Autodesk Fusion 360 part; units mm, degrees
(part 5 of 6)
  spline S26 degree 5 poles (0.4699, -23.4876) (0.4701, -23.4979) (0.4708, -23.5184) (0.4725, -23.5492) (0.4763, -23.5901) (0.4831, -23.6411) (0.4912, -23.692) (0.5002, -23.7429) (0.5098, -23.7937) (0.5196, -23.8445) (0.5298, -23.8953) (0.5405, -23.9461) (0.5517, -23.9968) (0.5636, -24.0474) (0.5762, -24.098) (0.5894, -24.1485) (0.6032, -24.1989) (0.6175, -24.2493) (0.6321, -24.2997) (0.6472, -24.35) (0.6626, -24.4003) (0.6784, -24.4505) (0.6946, -24.5006) (0.7112, -24.5507) (0.7283, -24.6008) (0.7458, -24.6508) (0.7636, -24.7007) (0.7819, -24.7506) (0.8005, -24.8004) (0.8194, -24.8502) (0.8387, -24.8999) (0.8583, -24.9496) (0.8782, -24.9992) (0.8985, -25.0487) (0.9191, -25.0982) (0.9401, -25.1476) (0.9614, -25.197) (0.983, -25.2463) (1.0049, -25.2956) (1.0272, -25.3448) (1.0497, -25.3939) (1.0725, -25.443) (1.0957, -25.492) (1.1191, -25.5409) (1.1429, -25.5898) (1.1669, -25.6386) (1.1912, -25.6874) (1.2158, -25.7361) (1.2407, -25.7847) (1.2659, -25.8333) (1.2913, -25.8818) (1.317, -25.9303) (1.343, -25.9787) (1.3693, -26.027) (1.3958, -26.0752) (1.4226, -26.1234) (1.4497, -26.1715) (1.477, -26.2196) (1.5046, -26.2675) (1.5325, -26.3154) (1.5606, -26.3633) (1.589, -26.4111) (1.6176, -26.4588) (1.6465, -26.5064) (1.6756, -26.5539) (1.705, -26.6014) (1.7346, -26.6489) (1.7645, -26.6962) (1.7946, -26.7435) (1.8249, -26.7907) (1.8555, -26.8378) (1.8802, -26.8754) (1.8988, -26.9036) (1.9113, -26.9224) (1.9175, -26.9318) knots 0 0 0 0 0 0 0.01428571 0.02857143 0.04285714 0.05714286 0.07142857 0.08571429 0.1 0.11428571 0.12857143 0.14285714 0.15714286 0.17142857 0.18571429 0.2 0.21428571 0.22857143 0.24285714 0.25714286 0.27142857 0.28571429 0.3 0.31428571 0.32857143 0.34285714 0.35714286 0.37142857 0.38571429 0.4 0.41428571 0.42857143 0.44285714 0.45714286 0.47142857 0.48571429 0.5 0.51428571 0.52857143 0.54285714 0.55714286 0.57142857 0.58571429 0.6 0.61428571 0.62857143 0.64285714 0.65714286 0.67142857 0.68571429 0.7 0.71428571 0.72857143 0.74285714 0.75714286 0.77142857 0.78571429 0.8 0.81428571 0.82857143 0.84285714 0.85714286 0.87142857 0.88571429 0.9 0.91428571 0.92857143 0.94285714 0.95714286 0.97142857 0.98571429 1 1 1 1 1 1
  arc A60 (1.9175, -26.9318) -> (3.3501, -26.7914) centre (0, 0) ccw
  spline S27 degree 5 poles (3.3501, -26.7914) (3.3544, -26.7809) (3.363, -26.7601) (3.3757, -26.7288) (3.3926, -26.6871) (3.4135, -26.6349) (3.4341, -26.5827) (3.4545, -26.5305) (3.4746, -26.4783) (3.4944, -26.426) (3.514, -26.3737) (3.5333, -26.3214) (3.5524, -26.269) (3.5712, -26.2167) (3.5898, -26.1643) (3.6081, -26.1119) (3.6261, -26.0595) (3.6438, -26.0071) (3.6613, -25.9547) (3.6785, -25.9022) (3.6955, -25.8497) (3.7121, -25.7972) (3.7285, -25.7448) (3.7446, -25.6922) (3.7604, -25.6397) (3.776, -25.5872) (3.7912, -25.5347) (3.8062, -25.4821) (3.8209, -25.4296) (3.8352, -25.377) (3.8493, -25.3244) (3.8631, -25.2719) (3.8766, -25.2193) (3.8898, -25.1667) (3.9027, -25.1142) (3.9152, -25.0616) (3.9275, -25.009) (3.9394, -24.9564) (3.951, -24.9039) (3.9623, -24.8513) (3.9733, -24.7987) (3.9839, -24.7462) (3.9942, -24.6936) (4.0041, -24.6411) (4.0137, -24.5886) (4.023, -24.5361) (4.0319, -24.4836) (4.0404, -24.4311) (4.0486, -24.3786) (4.0564, -24.3261) (4.0639, -24.2737) (4.0709, -24.2213) (4.0775, -24.1689) (4.0837, -24.1166) (4.0894, -24.0642) (4.0948, -24.012) (4.0997, -23.9597) (4.1043, -23.9074) (4.1085, -23.8552) (4.1122, -23.8031) (4.1154, -23.7509) (4.118, -23.6989) (4.1198, -23.6469) (4.121, -23.595) (4.1216, -23.5431) (4.1217, -23.4913) (4.1215, -23.4396) (4.121, -23.3879) (4.12, -23.3362) (4.1181, -23.2847) (4.1147, -23.2334) (4.1105, -23.1925) (4.1063, -23.162) (4.103, -23.1417) (4.1012, -23.1316) knots -1 -1 -1 -1 -1 -1 -0.98571429 -0.97142857 -0.95714286 -0.94285714 -0.92857143 -0.91428571 -0.9 -0.88571429 -0.87142857 -0.85714286 -0.84285714 -0.82857143 -0.81428571 -0.8 -0.78571429 -0.77142857 -0.75714286 -0.74285714 -0.72857143 -0.71428571 -0.7 -0.68571429 -0.67142857 -0.65714286 -0.64285714 -0.62857143 -0.61428571 -0.6 -0.58571429 -0.57142857 -0.55714286 -0.54285714 -0.52857143 -0.51428571 -0.5 -0.48571429 -0.47142857 -0.45714286 -0.44285714 -0.42857143 -0.41428571 -0.4 -0.38571429 -0.37142857 -0.35714286 -0.34285714 -0.32857143 -0.31428571 -0.3 -0.28571429 -0.27142857 -0.25714286 -0.24285714 -0.22857143 -0.21428571 -0.2 -0.18571429 -0.17142857 -0.15714286 -0.14285714 -0.12857143 -0.11428571 -0.1 -0.08571429 -0.07142857 -0.05714286 -0.04285714 -0.02857143 -0.01428571 0 0 0 0 0 0
  line L29 (4.1012, -23.1316) -> (4.0146, -22.641)
  arc A61 (4.409, -22.0638) -> (4.0146, -22.641) centre (4.507, -22.5541) ccw
  arc A62 (4.409, -22.0638) -> (5.5573, -21.8029) centre (0, 0) ccw
  arc A63 (6.1624, -22.153) -> (5.5573, -21.8029) centre (5.6808, -22.2874) ccw
  line L30 (6.1624, -22.153) -> (6.2962, -22.6329)
  spline S28 degree 5 poles (6.2962, -22.6329) (6.299, -22.6428) (6.3048, -22.6625) (6.3141, -22.6918) (6.328, -22.7305) (6.3472, -22.7783) (6.3677, -22.8255) (6.3891, -22.8725) (6.411, -22.9194) (6.4332, -22.9662) (6.4557, -23.0128) (6.4786, -23.0593) (6.5021, -23.1057) (6.5262, -23.1517) (6.551, -23.1976) (6.5764, -23.2432) (6.6023, -23.2887) (6.6287, -23.3339) (6.6554, -23.3791) (6.6824, -23.424) (6.7099, -23.4689) (6.7376, -23.5136) (6.7658, -23.5582) (6.7944, -23.6025) (6.8234, -23.6468) (6.8527, -23.6908) (6.8825, -23.7348) (6.9125, -23.7785) (6.9429, -23.8222) (6.9736, -23.8657) (7.0047, -23.9091) (7.036, -23.9523) (7.0677, -23.9954) (7.0996, -24.0383) (7.1319, -24.0811) (7.1645, -24.1238) (7.1974, -24.1663) (7.2306, -24.2087) (7.2641, -24.2509) (7.2979, -24.2931) (7.3319, -24.335) (7.3662, -24.3769) (7.4009, -24.4186) (7.4357, -24.4602) (7.4709, -24.5016) (7.5063, -24.543) (7.542, -24.5842) (7.5779, -24.6252) (7.6141, -24.6661) (7.6506, -24.7069) (7.6873, -24.7476) (7.7242, -24.7881) (7.7615, -24.8285) (7.7989, -24.8688) (7.8366, -24.9089) (7.8746, -24.9489) (7.9128, -24.9888) (7.9512, -25.0285) (7.9898, -25.0681) (8.0287, -25.1076) (8.0679, -25.1469) (8.1072, -25.1861) (8.1468, -25.2252) (8.1866, -25.2642) (8.2267, -25.303) (8.2669, -25.3417) (8.3074, -25.3803) (8.3481, -25.4187) (8.389, -25.457) (8.4302, -25.4952) (8.4715, -25.5332) (8.5048, -25.5635) (8.5298, -25.5862) (8.5466, -25.6013) (8.5549, -25.6088) knots 0 0 0 0 0 0 0.01428571 0.02857143 0.04285714 0.05714286 0.07142857 0.08571429 0.1 0.11428571 0.12857143 0.14285714 0.15714286 0.17142857 0.18571429 0.2 0.21428571 0.22857143 0.24285714 0.25714286 0.27142857 0.28571429 0.3 0.31428571 0.32857143 0.34285714 0.35714286 0.37142857 0.38571429 0.4 0.41428571 0.42857143 0.44285714 0.45714286 0.47142857 0.48571429 0.5 0.51428571 0.52857143 0.54285714 0.55714286 0.57142857 0.58571429 0.6 0.61428571 0.62857143 0.64285714 0.65714286 0.67142857 0.68571429 0.7 0.71428571 0.72857143 0.74285714 0.75714286 0.77142857 0.78571429 0.8 0.81428571 0.82857143 0.84285714 0.85714286 0.87142857 0.88571429 0.9 0.91428571 0.92857143 0.94285714 0.95714286 0.97142857 0.98571429 1 1 1 1 1 1
  arc A64 (8.5549, -25.6088) -> (9.9076, -25.1165) centre (0, 0) ccw
  spline S29 degree 5 poles (9.9076, -25.1165) (9.9092, -25.1054) (9.9123, -25.083) (9.9169, -25.0496) (9.9229, -25.005) (9.9301, -24.9492) (9.9371, -24.8935) (9.9438, -24.8379) (9.9503, -24.7823) (9.9565, -24.7267) (9.9625, -24.6712) (9.9682, -24.6157) (9.9736, -24.5603) (9.9789, -24.5049) (9.9838, -24.4496) (9.9885, -24.3943) (9.9929, -24.339) (9.9971, -24.2839) (10.0009, -24.2287) (10.0046, -24.1736) (10.0079, -24.1186) (10.011, -24.0636) (10.0138, -24.0087) (10.0164, -23.9538) (10.0186, -23.899) (10.0206, -23.8443) (10.0223, -23.7896) (10.0238, -23.735) (10.0249, -23.6804) (10.0258, -23.626) (10.0263, -23.5715) (10.0266, -23.5172) (10.0266, -23.4629) (10.0263, -23.4087) (10.0257, -23.3546) (10.0248, -23.3005) (10.0236, -23.2466) (10.0221, -23.1927) (10.0202, -23.1389) (10.0181, -23.0852) (10.0157, -23.0315) (10.0129, -22.978) (10.0098, -22.9245) (10.0063, -22.8712) (10.0026, -22.8179) (9.9985, -22.7647) (9.994, -22.7117) (9.9893, -22.6587) (9.9841, -22.6059) (9.9787, -22.5531) (9.9728, -22.5005) (9.9666, -22.448) (9.96, -22.3956) (9.9529, -22.3433) (9.9455, -22.2912) (9.9376, -22.2392) (9.9295, -22.1874) (9.9209, -22.1356) (9.912, -22.084) (9.9026, -22.0326) (9.8927, -21.9813) (9.8823, -21.9302) (9.8711, -21.8794) (9.8593, -21.8289) (9.847, -21.7785) (9.8343, -21.7283) (9.8212, -21.6782) (9.8078, -21.6282) (9.794, -21.5785) (9.7794, -21.529) (9.7634, -21.4801) (9.7491, -21.4416) (9.7374, -21.4131) (9.7292, -21.3943) (9.7249, -21.3849) knots -1 -1 -1 -1 -1 -1 -0.98571429 -0.97142857 -0.95714286 -0.94285714 -0.92857143 -0.91428571 -0.9 -0.88571429 -0.87142857 -0.85714286 -0.84285714 -0.82857143 -0.81428571 -0.8 -0.78571429 -0.77142857 -0.75714286 -0.74285714 -0.72857143 -0.71428571 -0.7 -0.68571429 -0.67142857 -0.65714286 -0.64285714 -0.62857143 -0.61428571 -0.6 -0.58571429 -0.57142857 -0.55714286 -0.54285714 -0.52857143 -0.51428571 -0.5 -0.48571429 -0.47142857 -0.45714286 -0.44285714 -0.42857143 -0.41428571 -0.4 -0.38571429 -0.37142857 -0.35714286 -0.34285714 -0.32857143 -0.31428571 -0.3 -0.28571429 -0.27142857 -0.25714286 -0.24285714 -0.22857143 -0.21428571 -0.2 -0.18571429 -0.17142857 -0.15714286 -0.14285714 -0.12857143 -0.11428571 -0.1 -0.08571429 -0.07142857 -0.05714286 -0.04285714 -0.02857143 -0.01428571 0 0 0 0 0 0
  line L31 (9.7249, -21.3849) -> (9.5191, -20.9313)
  arc A65 (9.7575, -20.2741) -> (9.5191, -20.9313) centre (9.9744, -20.7247) ccw
  arc A66 (9.7575, -20.2741) -> (10.8048, -19.7359) centre (0, 0) ccw
  arc A67 (11.478, -19.9245) -> (10.8048, -19.7359) centre (11.0449, -20.1745) ccw
  line L32 (11.478, -19.9245) -> (11.727, -20.356)
  spline S30 degree 5 poles (11.727, -20.356) (11.7321, -20.3649) (11.7426, -20.3826) (11.759, -20.4087) (11.782, -20.4427) (11.8125, -20.4842) (11.8442, -20.5248) (11.8766, -20.565) (11.9094, -20.605) (11.9425, -20.6448) (11.9759, -20.6844) (12.0097, -20.7237) (12.044, -20.7627) (12.0788, -20.8014) (12.1142, -20.8396) (12.1501, -20.8775) (12.1865, -20.9151) (12.2233, -20.9524) (12.2604, -20.9894) (12.2978, -21.0263) (12.3355, -21.0629) (12.3736, -21.0993) (12.4119, -21.1354) (12.4507, -21.1713) (12.4897, -21.207) (12.5291, -21.2423) (12.5688, -21.2775) (12.6088, -21.3124) (12.6491, -21.3471) (12.6897, -21.3816) (12.7305, -21.4159) (12.7716, -21.45) (12.813, -21.4838) (12.8547, -21.5175) (12.8966, -21.5509) (12.9388, -21.5841) (12.9812, -21.6171) (13.0239, -21.6499) (13.0669, -21.6825) (13.11, -21.7149) (13.1535, -21.7471) (13.1971, -21.7791) (13.241, -21.8109) (13.2851, -21.8425) (13.3295, -21.874) (13.3741, -21.9052) (13.4189, -21.9362) (13.4639, -21.967) (13.5091, -21.9976) (13.5546, -22.0281) (13.6002, -22.0583) (13.6461, -22.0884) (13.6922, -22.1183) (13.7385, -22.1479) (13.785, -22.1774) (13.8317, -22.2067) (13.8786, -22.2359) (13.9257, -22.2648) (13.973, -22.2935) (14.0205, -22.3221) (14.0682, -22.3505) (14.1161, -22.3787) (14.1641, -22.4067) (14.2124, -22.4345) (14.2608, -22.4622) (14.3094, -22.4896) (14.3582, -22.5169) (14.4072, -22.544) (14.4564, -22.5709) (14.5057, -22.5977) (14.5552, -22.6242) (14.595, -22.6453) (14.6249, -22.6611) (14.6448, -22.6716) (14.6548, -22.6768) knots 0 0 0 0 0 0 0.01428571 0.02857143 0.04285714 0.05714286 0.07142857 0.08571429 0.1 0.11428571 0.12857143 0.14285714 0.15714286 0.17142857 0.18571429 0.2 0.21428571 0.22857143 0.24285714 0.25714286 0.27142857 0.28571429 0.3 0.31428571 0.32857143 0.34285714 0.35714286 0.37142857 0.38571429 0.4 0.41428571 0.42857143 0.44285714 0.45714286 0.47142857 0.48571429 0.5 0.51428571 0.52857143 0.54285714 0.55714286 0.57142857 0.58571429 0.6 0.61428571 0.62857143 0.64285714 0.65714286 0.67142857 0.68571429 0.7 0.71428571 0.72857143 0.74285714 0.75714286 0.77142857 0.78571429 0.8 0.81428571 0.82857143 0.84285714 0.85714286 0.87142857 0.88571429 0.9 0.91428571 0.92857143 0.94285714 0.95714286 0.97142857 0.98571429 1 1 1 1 1 1
  arc A68 (14.6548, -22.6768) -> (15.8426, -21.8635) centre (0, 0) ccw
  spline S31 degree 5 poles (15.8426, -21.8635) (15.8413, -21.8523) (15.8388, -21.8299) (15.8349, -21.7964) (15.8296, -21.7517) (15.8227, -21.6959) (15.8156, -21.6402) (15.8083, -21.5847) (15.8008, -21.5292) (15.793, -21.4738) (15.785, -21.4186) (15.7767, -21.3634) (15.7682, -21.3084) (15.7595, -21.2534) (15.7505, -21.1986) (15.7413, -21.1439) (15.7318, -21.0893) (15.7221, -21.0348) (15.7122, -20.9804) (15.702, -20.9261) (15.6916, -20.872) (15.6809, -20.818) (15.6699, -20.7641) (15.6588, -20.7103) (15.6473, -20.6567) (15.6356, -20.6031) (15.6237, -20.5498) (15.6115, -20.4965) (15.599, -20.4434) (15.5863, -20.3904) (15.5733, -20.3375) (15.5601, -20.2848) (15.5466, -20.2323) (15.5328, -20.1799) (15.5188, -20.1276) (15.5044, -20.0755) (15.4898, -20.0235) (15.475, -19.9717) (15.4598, -19.92) (15.4444, -19.8685) (15.4287, -19.8171) (15.4127, -19.766) (15.3964, -19.715) (15.3798, -19.6641) (15.3629, -19.6135) (15.3457, -19.563) (15.3282, -19.5127) (15.3104, -19.4626) (15.2923, -19.4127) (15.2739, -19.363) (15.2552, -19.3134) (15.2361, -19.2641) (15.2166, -19.215) (15.1968, -19.1662) (15.1766, -19.1176) (15.1561, -19.0692) (15.1353, -19.021) (15.1141, -18.973) (15.0927, -18.9252) (15.0708, -18.8777) (15.0485, -18.8305) (15.0256, -18.7837) (15.0022, -18.7372) (14.9782, -18.6911) (14.9537, -18.6454) (14.9289, -18.6) (14.9038, -18.5547) (14.8784, -18.5096) (14.8527, -18.4649) (14.8262, -18.4206) (14.7985, -18.3773) (14.7752, -18.3435) (14.7567, -18.3188) (14.7441, -18.3026) (14.7376, -18.2946) knots -1 -1 -1 -1 -1 -1 -0.98571429 -0.97142857 -0.95714286 -0.94285714 -0.92857143 -0.91428571 -0.9 -0.88571429 -0.87142857 -0.85714286 -0.84285714 -0.82857143 -0.81428571 -0.8 -0.78571429 -0.77142857 -0.75714286 -0.74285714 -0.72857143 -0.71428571 -0.7 -0.68571429 -0.67142857 -0.65714286 -0.64285714 -0.62857143 -0.61428571 -0.6 -0.58571429 -0.57142857 -0.55714286 -0.54285714 -0.52857143 -0.51428571 -0.5 -0.48571429 -0.47142857 -0.45714286 -0.44285714 -0.42857143 -0.41428571 -0.4 -0.38571429 -0.37142857 -0.35714286 -0.34285714 -0.32857143 -0.31428571 -0.3 -0.28571429 -0.27142857 -0.25714286 -0.24285714 -0.22857143 -0.21428571 -0.2 -0.18571429 -0.17142857 -0.15714286 -0.14285714 -0.12857143 -0.11428571 -0.1 -0.08571429 -0.07142857 -0.05714286 -0.04285714 -0.02857143 -0.01428571 0 0 0 0 0 0
  line L33 (14.7376, -18.2946) -> (14.4254, -17.9064)
  arc A69 (14.493, -17.2106) -> (14.4254, -17.9064) centre (14.815, -17.593) ccw
  arc A70 (14.493, -17.2106) -> (15.3735, -16.4288) centre (0, 0) ccw
  arc A71 (16.0724, -16.4441) -> (15.3735, -16.4288) centre (15.7151, -16.7939) ccw
  line L34 (16.0724, -16.4441) -> (16.4209, -16.8001)
  spline S32 degree 5 poles (16.4209, -16.8001) (16.4281, -16.8074) (16.4426, -16.8219) (16.465, -16.8432) (16.4958, -16.8704) (16.5356, -16.903) (16.5764, -16.9345) (16.6178, -16.9654) (16.6595, -16.9959) (16.7015, -17.0262) (16.7437, -17.0562) (16.7862, -17.0859) (16.8291, -17.1152) (16.8724, -17.144) (16.9162, -17.1722) (16.9605, -17.2) (17.005, -17.2273) (17.0499, -17.2543) (17.0951, -17.281) (17.1405, -17.3074) (17.1861, -17.3335) (17.232, -17.3592) (17.2782, -17.3847) (17.3246, -17.4098) (17.3713, -17.4346) (17.4183, -17.4591) (17.4655, -17.4833) (17.5129, -17.5072) (17.5606, -17.5308) (17.6084, -17.5541) (17.6565, -17.5771) (17.7048, -17.5999) (17.7533, -17.6224) (17.802, -17.6446) (17.8509, -17.6666) (17.9, -17.6883) (17.9494, -17.7097) (17.9989, -17.7308) (18.0486, -17.7517) (18.0984, -17.7724) (18.1485, -17.7928) (18.1988, -17.8129) (18.2492, -17.8328) (18.2998, -17.8524) (18.3505, -17.8718) (18.4015, -17.891) (18.4526, -17.9099) (18.5039, -17.9285) (18.5553, -17.947) (18.6069, -17.9651) (18.6587, -17.9831) (18.7106, -18.0008) (18.7626, -18.0183) (18.8149, -18.0355) (18.8672, -18.0525) (18.9198, -18.0693) (18.9724, -18.0858) (19.0252, -18.1021) (19.0782, -18.1182) (19.1313, -18.1341) (19.1845, -18.1497) (19.2379, -18.1651) (19.2914, -18.1803) (19.3451, -18.1952) (19.3989, -18.21) (19.4528, -18.2245) (19.5069, -18.2388) (19.561, -18.2528) (19.6154, -18.2667) (19.6698, -18.2803) (19.7244, -18.2937) (19.7681, -18.3043) (19.801, -18.3121) (19.8229, -18.3173) (19.8339, -18.3198) knots 0 0 0 0 0 0 0.01428571 0.02857143 0.04285714 0.05714286 0.07142857 0.08571429 0.1 0.11428571 0.12857143 0.14285714 0.15714286 0.17142857 0.18571429 0.2 0.21428571 0.22857143 0.24285714 0.25714286 0.27142857 0.28571429 0.3 0.31428571 0.32857143 0.34285714 0.35714286 0.37142857 0.38571429 0.4 0.41428571 0.42857143 0.44285714 0.45714286 0.47142857 0.48571429 0.5 0.51428571 0.52857143 0.54285714 0.55714286 0.57142857 0.58571429 0.6 0.61428571 0.62857143 0.64285714 0.65714286 0.67142857 0.68571429 0.7 0.71428571 0.72857143 0.74285714 0.75714286 0.77142857 0.78571429 0.8 0.81428571 0.82857143 0.84285714 0.85714286 0.87142857 0.88571429 0.9 0.91428571 0.92857143 0.94285714 0.95714286 0.97142857 0.98571429 1 1 1 1 1 1
  arc A72 (19.8339, -18.3198) -> (20.7821, -17.2368) centre (0, 0) ccw
  spline S33 degree 5 poles (20.7821, -17.2368) (20.7781, -17.2262) (20.77, -17.2052) (20.7579, -17.1736) (20.7417, -17.1316) (20.7212, -17.0793) (20.7005, -17.0272) (20.6796, -16.9752) (20.6585, -16.9233) (20.6371, -16.8716) (20.6156, -16.8201) (20.5939, -16.7687) (20.572, -16.7175) (20.5499, -16.6665) (20.5275, -16.6156) (20.505, -16.5649) (20.4823, -16.5144) (20.4593, -16.464) (20.4362, -16.4138) (20.4128, -16.3638) (20.3892, -16.3139) (20.3654, -16.2643) (20.3415, -16.2148) (20.3173, -16.1655) (20.2928, -16.1164) (20.2682, -16.0674) (20.2434, -16.0187) (20.2183, -15.9701) (20.193, -15.9218) (20.1675, -15.8736) (20.1418, -15.8257) (20.1159, -15.7779) (20.0897, -15.7304) (20.0633, -15.683) (20.0367, -15.6359) (20.0099, -15.5889) (19.9828, -15.5422) (19.9556, -15.4957) (19.928, -15.4495) (19.9003, -15.4034) (19.8723, -15.3576) (19.8441, -15.312) (19.8156, -15.2667) (19.7869, -15.2216) (19.7579, -15.1767) (19.7287, -15.1321) (19.6993, -15.0877) (19.6696, -15.0436) (19.6396, -14.9998) (19.6094, -14.9562) (19.5789, -14.9129) (19.5482, -14.8698) (19.5171, -14.8272) (19.4858, -14.7848) (19.4542, -14.7427) (19.4223, -14.7009) (19.3901, -14.6594) (19.3577, -14.6182) (19.325, -14.5772) (19.292, -14.5367) (19.2587, -14.4965) (19.2249, -14.4568) (19.1906, -14.4176) (19.1559, -14.379) (19.1209, -14.3408) (19.0855, -14.3029) (19.0499, -14.2653) (19.0141, -14.228) (18.9781, -14.1911) (18.9414, -14.1548) (18.9039, -14.1197) (18.8728, -14.0927) (18.8488, -14.0734) (18.8325, -14.0609) (18.8243, -14.0547) knots -1 -1 -1 -1 -1 -1 -0.98571429 -0.97142857 -0.95714286 -0.94285714 -0.92857143 -0.91428571 -0.9 -0.88571429 -0.87142857 -0.85714286 -0.84285714 -0.82857143 -0.81428571 -0.8 -0.78571429 -0.77142857 -0.75714286 -0.74285714 -0.72857143 -0.71428571 -0.7 -0.68571429 -0.67142857 -0.65714286 -0.64285714 -0.62857143 -0.61428571 -0.6 -0.58571429 -0.57142857 -0.55714286 -0.54285714 -0.52857143 -0.51428571 -0.5 -0.48571429 -0.47142857 -0.45714286 -0.44285714 -0.42857143 -0.41428571 -0.4 -0.38571429 -0.37142857 -0.35714286 -0.34285714 -0.32857143 -0.31428571 -0.3 -0.28571429 -0.27142857 -0.25714286 -0.24285714 -0.22857143 -0.21428571 -0.2 -0.18571429 -0.17142857 -0.15714286 -0.14285714 -0.12857143 -0.11428571 -0.1 -0.08571429 -0.07142857 -0.05714286 -0.04285714 -0.02857143 -0.01428571 0 0 0 0 0 0
  line L35 (18.8243, -14.0547) -> (18.4253, -13.7564)
  arc A73 (18.3177, -13.0656) -> (18.4253, -13.7564) centre (18.7248, -13.356) ccw
  arc A74 (18.3177, -13.0656) -> (18.9762, -12.0894) centre (0, 0) ccw
  arc A75 (19.657, -11.9304) -> (18.9762, -12.0894) centre (19.3979, -12.3581) ccw
  line L36 (19.657, -11.9304) -> (20.083, -12.1886)
  spline S34 degree 5 poles (20.083, -12.1886) (20.0918, -12.1939) (20.1095, -12.2043) (20.1364, -12.2193) (20.173, -12.238) (20.2197, -12.2597) (20.267, -12.2801) (20.3148, -12.2997) (20.3628, -12.3189) (20.411, -12.3378) (20.4594, -12.3564) (20.5079, -12.3746) (20.5567, -12.3923) (20.6059, -12.4094) (20.6553, -12.4258) (20.7051, -12.4417) (20.7551, -12.4571) (20.8053, -12.4721) (20.8556, -12.4867) (20.9061, -12.501) (20.9568, -12.5149) (21.0077, -12.5284) (21.0587, -12.5416) (21.11, -12.5544) (21.1614, -12.5668) (21.2129, -12.5789) (21.2647, -12.5905) (21.3166, -12.6019) (21.3686, -12.6129) (21.4207, -12.6236) (21.473, -12.6339) (21.5255, -12.644) (21.5781, -12.6537) (21.6308, -12.6631) (21.6836, -12.6722) (21.7366, -12.681) (21.7897, -12.6895) (21.8429, -12.6977) (21.8962, -12.7055) (21.9497, -12.7131) (22.0032, -12.7204) (22.0569, -12.7274) (22.1107, -12.7342) (22.1646, -12.7406) (22.2186, -12.7468) (22.2727, -12.7526) (22.3269, -12.7582) (22.3812, -12.7636) (22.4356, -12.7686) (22.4901, -12.7734) (22.5447, -12.7779) (22.5994, -12.7821) (22.6541, -12.7861) (22.709, -12.7898) (22.764, -12.7933) (22.819, -12.7964) (22.8741, -12.7994) (22.9293, -12.802) (22.9846, -12.8044) (23.04, -12.8066) (23.0955, -12.8085) (23.151, -12.8101) (23.2066, -12.8115) (23.2623, -12.8127) (23.3181, -12.8136) (23.3739, -12.8142) (23.4298, -12.8146) (23.4858, -12.8148) (23.5418, -12.8147) (23.598, -12.8143) (23.6541, -12.8137) (23.6992, -12.8131) (23.7329, -12.8125) (23.7555, -12.812) (23.7667, -12.8118) knots 0 0 0 0 0 0 0.01428571 0.02857143 0.04285714 0.05714286 0.07142857 0.08571429 0.1 0.11428571 0.12857143 0.14285714 0.15714286 0.17142857 0.18571429 0.2 0.21428571 0.22857143 0.24285714 0.25714286 0.27142857 0.28571429 0.3 0.31428571 0.32857143 0.34285714 0.35714286 0.37142857 0.38571429 0.4 0.41428571 0.42857143 0.44285714 0.45714286 0.47142857 0.48571429 0.5 0.51428571 0.52857143 0.54285714 0.55714286 0.57142857 0.58571429 0.6 0.61428571 0.62857143 0.64285714 0.65714286 0.67142857 0.68571429 0.7 0.71428571 0.72857143 0.74285714 0.75714286 0.77142857 0.78571429 0.8 0.81428571 0.82857143 0.84285714 0.85714286 0.87142857 0.88571429 0.9 0.91428571 0.92857143 0.94285714 0.95714286 0.97142857 0.98571429 1 1 1 1 1 1
  arc A76 (23.7667, -12.8118) -> (24.4158, -11.5269) centre (0, 0) ccw
  spline S35 degree 5 poles (24.4158, -11.5269) (24.4093, -11.5177) (24.3963, -11.4993) (24.3767, -11.4718) (24.3505, -11.4352) (24.3176, -11.3896) (24.2846, -11.3442) (24.2514, -11.2991) (24.2181, -11.2541) (24.1846, -11.2093) (24.1509, -11.1648) (24.1171, -11.1204) (24.0832, -11.0763) (24.049, -11.0323) (24.0148, -10.9886) (23.9803, -10.9451) (23.9457, -10.9018) (23.911, -10.8587) (23.8761, -10.8159) (23.841, -10.7732) (23.8058, -10.7308) (23.7704, -10.6886) (23.7348, -10.6467) (23.6991, -10.6049) (23.6633, -10.5634) (23.6273, -10.5222) (23.5911, -10.4811) (23.5547, -10.4403) (23.5182, -10.3998) (23.4815, -10.3595) (23.4447, -10.3194) (23.4077, -10.2796) (23.3706, -10.2401) (23.3332, -10.2008) (23.2957, -10.1617) (23.2581, -10.1229) (23.2202, -10.0844) (23.1823, -10.0462) (23.1441, -10.0082) (23.1058, -9.9705) (23.0673, -9.9331) (23.0286, -9.8959) (22.9897, -9.8591) (22.9507, -9.8226) (22.9115, -9.7863) (22.8721, -9.7504) (22.8325, -9.7147) (22.7928, -9.6794) (22.7529, -9.6443) (22.7128, -9.6096) (22.6725, -9.5753) (22.632, -9.5412) (22.5913, -9.5076) (22.5504, -9.4744) (22.5093, -9.4415) (22.468, -9.4089) (22.4266, -9.3767) (22.3849, -9.3449) (22.3431, -9.3133) (22.301, -9.2822) (22.2587, -9.2516) (22.2161, -9.2216) (22.1732, -9.1922) (22.13, -9.1634) (22.0866, -9.1351) (22.0429, -9.1072) (21.9991, -9.0797) (21.9551, -9.0524) (21.911, -9.0256) (21.8665, -8.9996) (21.8214, -8.9749) (21.7846, -8.9565) (21.7566, -8.9437) (21.7377, -8.9357) (21.7281, -8.9318) knots -1 -1 -1 -1 -1 -1 -0.98571429 -0.97142857 -0.95714286 -0.94285714 -0.92857143 -0.91428571 -0.9 -0.88571429 -0.87142857 -0.85714286 -0.84285714 -0.82857143 -0.81428571 -0.8 -0.78571429 -0.77142857 -0.75714286 -0.74285714 -0.72857143 -0.71428571 -0.7 -0.68571429 -0.67142857 -0.65714286 -0.64285714 -0.62857143 -0.61428571 -0.6 -0.58571429 -0.57142857 -0.55714286 -0.54285714 -0.52857143 -0.51428571 -0.5 -0.48571429 -0.47142857 -0.45714286 -0.44285714 -0.42857143 -0.41428571 -0.4 -0.38571429 -0.37142857 -0.35714286 -0.34285714 -0.32857143 -0.31428571 -0.3 -0.28571429 -0.27142857 -0.25714286 -0.24285714 -0.22857143 -0.21428571 -0.2 -0.18571429 -0.17142857 -0.15714286 -0.14285714 -0.12857143 -0.11428571 -0.1 -0.08571429 -0.07142857 -0.05714286 -0.04285714 -0.02857143 -0.01428571 0 0 0 0 0 0
  line L37 (21.7281, -8.9318) -> (21.2676, -8.742)
  arc A77 (20.9915, -8.0997) -> (21.2676, -8.742) centre (21.458, -8.2797) ccw
  arc A78 (20.9915, -8.0997) -> (21.3865, -6.9904) centre (0, 0) ccw
  arc A79 (22.0064, -6.6671) -> (21.3865, -6.9904) centre (21.8618, -7.1458) ccw
  line L38 (22.0064, -6.6671) -> (22.4832, -6.8112)
  spline S36 degree 5 poles (22.4832, -6.8112) (22.4931, -6.8142) (22.5128, -6.8199) (22.5426, -6.8277) (22.5827, -6.8367) (22.6333, -6.8461) (22.6842, -6.8541) (22.7354, -6.8612) (22.7867, -6.8678) (22.838, -6.8742) (22.8895, -6.8802) (22.9411, -6.8857) (22.9928, -6.8907) (23.0446, -6.895) (23.0966, -6.8987) (23.1487, -6.9017) (23.201, -6.9042) (23.2533, -6.9062) (23.3057, -6.9078) (23.3582, -6.9091) (23.4108, -6.9099) (23.4634, -6.9104) (23.5161, -6.9105) (23.5689, -6.9102) (23.6218, -6.9094) (23.6747, -6.9082) (23.7277, -6.9067) (23.7808, -6.9047) (23.8339, -6.9025) (23.8871, -6.8998) (23.9404, -6.8969) (23.9937, -6.8936) (24.047, -6.8899) (24.1004, -6.8859) (24.1538, -6.8816) (24.2073, -6.8769) (24.2609, -6.8719) (24.3144, -6.8666) (24.368, -6.861) (24.4217, -6.8551) (24.4754, -6.8488) (24.5291, -6.8423) (24.5829, -6.8354) (24.6367, -6.8282) (24.6905, -6.8208) (24.7444, -6.813) (24.7983, -6.8049) (24.8522, -6.7966) (24.9061, -6.788) (24.9601, -6.779) (25.0141, -6.7698) (25.0681, -6.7603) (25.1222, -6.7506) (25.1762, -6.7405) (25.2303, -6.7302) (25.2844, -6.7196) (25.3386, -6.7087) (25.3927, -6.6975) (25.4469, -6.6861) (25.501, -6.6744) (25.5552, -6.6625) (25.6094, -6.6503) (25.6636, -6.6378) (25.7179, -6.625) (25.7721, -6.612) (25.8263, -6.5988) (25.8806, -6.5852) (25.9348, -6.5715) (25.9891, -6.5574) (26.0434, -6.5432) (26.0977, -6.5286) (26.1411, -6.5168) (26.1737, -6.5078) (26.1954, -6.5018) (26.2062, -6.4987) knots 0 0 0 0 0 0 0.01428571 0.02857143 0.04285714 0.05714286 0.07142857 0.08571429 0.1 0.11428571 0.12857143 0.14285714 0.15714286 0.17142857 0.18571429 0.2 0.21428571 0.22857143 0.24285714 0.25714286 0.27142857 0.28571429 0.3 0.31428571 0.32857143 0.34285714 0.35714286 0.37142857 0.38571429 0.4 0.41428571 0.42857143 0.44285714 0.45714286 0.47142857 0.48571429 0.5 0.51428571 0.52857143 0.54285714 0.55714286 0.57142857 0.58571429 0.6 0.61428571 0.62857143 0.64285714 0.65714286 0.67142857 0.68571429 0.7 0.71428571 0.72857143 0.74285714 0.75714286 0.77142857 0.78571429 0.8 0.81428571 0.82857143 0.84285714 0.85714286 0.87142857 0.88571429 0.9 0.91428571 0.92857143 0.94285714 0.95714286 0.97142857 0.98571429 1 1 1 1 1 1
  arc A80 (26.2062, -6.4987) -> (26.5153, -5.0928) centre (0, 0) ccw
  spline S37 degree 5 poles (26.5153, -5.0928) (26.5067, -5.0855) (26.4896, -5.0709) (26.4638, -5.0491) (26.4293, -5.0202) (26.3861, -4.9842) (26.3429, -4.9485) (26.2995, -4.913) (26.256, -4.8777) (26.2124, -4.8427) (26.1688, -4.8079) (26.125, -4.7734) (26.0811, -4.739) (26.0371, -4.705) (25.993, -4.6711) (25.9489, -4.6376) (25.9046, -4.6042) (25.8602, -4.5712) (25.8158, -4.5383) (25.7712, -4.5057) (25.7265, -4.4734) (25.6817, -4.4414) (25.6369, -4.4096) (25.5919, -4.378) (25.5469, -4.3467) (25.5017, -4.3157) (25.4565, -4.285) (25.4111, -4.2545) (25.3657, -4.2243) (25.3201, -4.1944) (25.2745, -4.1647) (25.2288, -4.1354) (25.1829, -4.1063) (25.137, -4.0775) (25.091, -4.0491) (25.0448, -4.0209) (24.9986, -3.993) (24.9523, -3.9654) (24.9059, -3.9381) (24.8594, -3.9111) (24.8128, -3.8844) (24.7661, -3.8581) (24.7193, -3.832) (24.6724, -3.8064) (24.6254, -3.781) (24.5783, -3.756) (24.5312, -3.7313) (24.4839, -3.7069) (24.4365, -3.6829) (24.3891, -3.6593) (24.3415, -3.636) (24.2938, -3.6131) (24.246, -3.5907) (24.1981, -3.5686) (24.1502, -3.547) (24.1021, -3.5258) (24.0539, -3.5049) (24.0056, -3.4844) (23.9573, -3.4642) (23.9088, -3.4446) (23.8602, -3.4254) (23.8115, -3.4069) (23.7626, -3.3891) (23.7136, -3.372) (23.6645, -3.3554) (23.6152, -3.3393) (23.566, -3.3234) (23.5166, -3.308) (23.4672, -3.293) (23.4176, -3.2789) (23.3678, -3.2661) (23.3276, -3.2575) (23.2973, -3.2521) (23.2769, -3.249) (23.2668, -3.2476) knots -1 -1 -1 -1 -1 -1 -0.98571429 -0.97142857 -0.95714286 -0.94285714 -0.92857143 -0.91428571 -0.9 -0.88571429 -0.87142857 -0.85714286 -0.84285714 -0.82857143 -0.81428571 -0.8 -0.78571429 -0.77142857 -0.75714286 -0.74285714 -0.72857143 -0.71428571 -0.7 -0.68571429 -0.67142857 -0.65714286 -0.64285714 -0.62857143 -0.61428571 -0.6 -0.58571429 -0.57142857 -0.55714286 -0.54285714 -0.52857143 -0.51428571 -0.5 -0.48571429 -0.47142857 -0.45714286 -0.44285714 -0.42857143 -0.41428571 -0.4 -0.38571429 -0.37142857 -0.35714286 -0.34285714 -0.32857143 -0.31428571 -0.3 -0.28571429 -0.27142857 -0.25714286 -0.24285714 -0.22857143 -0.21428571 -0.2 -0.18571429 -0.17142857 -0.15714286 -0.14285714 -0.12857143 -0.11428571 -0.1 -0.08571429 -0.07142857 -0.05714286 -0.04285714 -0.02857143 -0.01428571 0 0 0 0 0 0
  line L39 (23.2668, -3.2476) -> (22.7734, -3.1783)
  arc A81 (22.3464, -2.6249) -> (22.7734, -3.1783) centre (22.843, -2.6832) ccw
  arc A82 (22.3464, -2.6249) -> (22.4531, -1.4522) centre (0, 0) ccw
  arc A83 (22.9731, -0.9849) -> (22.4531, -1.4522) centre (22.952, -1.4845) ccw
  line L40 (22.9731, -0.9849) -> (23.4708, -1.0059)
  spline S38 degree 5 poles (23.4708, -1.0059) (23.481, -1.0063) (23.5016, -1.0069) (23.5324, -1.0071) (23.5735, -1.0058) (23.6248, -1.0023) (23.6761, -0.9974) (23.7274, -0.9916) (23.7788, -0.9853) (23.8301, -0.9786) (23.8814, -0.9716) (23.9327, -0.9642) (23.984, -0.9562) (24.0353, -0.9475) (24.0866, -0.9381) (24.1378, -0.928) (24.1891, -0.9174) (24.2402, -0.9064) (24.2914, -0.8949) (24.3426, -0.8831) (24.3937, -0.8708) (24.4448, -0.8582) (24.4959, -0.8452) (24.5469, -0.8317) (24.598, -0.8178) (24.6489, -0.8035) (24.6999, -0.7888) (24.7508, -0.7738) (24.8017, -0.7584) (24.8526, -0.7426) (24.9034, -0.7265) (24.9542, -0.71) (25.005, -0.6932) (25.0557, -0.6761) (25.1064, -0.6586) (25.157, -0.6408) (25.2076, -0.6226) (25.2582, -0.6042) (25.3087, -0.5854) (25.3592, -0.5663) (25.4097, -0.5469) (25.4601, -0.5272) (25.5105, -0.5071) (25.5608, -0.4868) (25.6111, -0.4662) (25.6613, -0.4453) (25.7115, -0.4241) (25.7617, -0.4026) (25.8118, -0.3808) (25.8618, -0.3587) (25.9118, -0.3364) (25.9618, -0.3137) (26.0117, -0.2908) (26.0616, -0.2677) (26.1114, -0.2442) (26.1612, -0.2205) (26.2109, -0.1965) (26.2606, -0.1722) (26.3102, -0.1477) (26.3597, -0.1229) (26.4092, -0.0978) (26.4587, -0.0725) (26.5081, -0.047) (26.5575, -0.0211) (26.6068, 0.005) (26.656, 0.0313) (26.7052, 0.0579) (26.7543, 0.0847) (26.8034, 0.1118) (26.8524, 0.1391) (26.9014, 0.1667) (26.9405, 0.189) (26.9698, 0.2058) (26.9893, 0.217) (26.9991, 0.2227) knots 0 0 0 0 0 0 0.01428571 0.02857143 0.04285714 0.05714286 0.07142857 0.08571429 0.1 0.11428571 0.12857143 0.14285714 0.15714286 0.17142857 0.18571429 0.2 0.21428571 0.22857143 0.24285714 0.25714286 0.27142857 0.28571429 0.3 0.31428571 0.32857143 0.34285714 0.35714286 0.37142857 0.38571429 0.4 0.41428571 0.42857143 0.44285714 0.45714286 0.47142857 0.48571429 0.5 0.51428571 0.52857143 0.54285714 0.55714286 0.57142857 0.58571429 0.6 0.61428571 0.62857143 0.64285714 0.65714286 0.67142857 0.68571429 0.7 0.71428571 0.72857143 0.74285714 0.75714286 0.77142857 0.78571429 0.8 0.81428571 0.82857143 0.84285714 0.85714286 0.87142857 0.88571429 0.9 0.91428571 0.92857143 0.94285714 0.95714286 0.97142857 0.98571429 1 1 1 1 1 1
  arc A84 (26.9991, 0.2227) -> (26.9488, 1.6612) centre (0, 0) ccw
  spline S39 degree 5 poles (26.9488, 1.6612) (26.9387, 1.6662) (26.9184, 1.6761) (26.888, 1.6908) (26.8475, 1.7102) (26.7967, 1.7343) (26.7459, 1.7582) (26.6951, 1.7818) (26.6442, 1.8051) (26.5933, 1.8282) (26.5423, 1.851) (26.4913, 1.8736) (26.4403, 1.896) (26.3892, 1.918) (26.3381, 1.9398) (26.287, 1.9614) (26.2358, 1.9826) (26.1846, 2.0036) (26.1333, 2.0244) (26.0821, 2.0448) (26.0308, 2.065) (25.9794, 2.085) (25.9281, 2.1046) (25.8767, 2.124) (25.8253, 2.1431) (25.7738, 2.1619) (25.7223, 2.1804) (25.6708, 2.1986) (25.6193, 2.2166) (25.5677, 2.2342) (25.5162, 2.2516) (25.4646, 2.2687) (25.413, 2.2854) (25.3613, 2.3019) (25.3096, 2.318) (25.258, 2.3339) (25.2063, 2.3494) (25.1545, 2.3646) (25.1028, 2.3795) (25.051, 2.3941) (24.9993, 2.4083) (24.9475, 2.4222) (24.8957, 2.4358) (24.8439, 2.449) (24.7921, 2.4619) (24.7402, 2.4744) (24.6884, 2.4866) (24.6366, 2.4984) (24.5847, 2.5099) (24.5329, 2.521) (24.481, 2.5317) (24.4291, 2.542) (24.3773, 2.5519) (24.3254, 2.5613) (24.2735, 2.5703) (24.2217, 2.579) (24.1698, 2.5872) (24.118, 2.5951) (24.0661, 2.6025) (24.0143, 2.6095) (23.9625, 2.616) (23.9107, 2.6218) (23.8589, 2.6269) (23.8072, 2.6313) (23.7555, 2.6351) (23.7038, 2.6385) (23.6521, 2.6416) (23.6005, 2.6443) (23.5489, 2.6465) (23.4973, 2.6479) (23.4459, 2.6478) (23.4048, 2.6462) (23.3741, 2.6438) (23.3537, 2.6418) (23.3434, 2.6406) knots -1 -1 -1 -1 -1 -1 -0.98571429 -0.97142857 -0.95714286 -0.94285714 -0.92857143 -0.91428571 -0.9 -0.88571429 -0.87142857 -0.85714286 -0.84285714 -0.82857143 -0.81428571 -0.8 -0.78571429 -0.77142857 -0.75714286 -0.74285714 -0.72857143 -0.71428571 -0.7 -0.68571429 -0.67142857 -0.65714286 -0.64285714 -0.62857143 -0.61428571 -0.6 -0.58571429 -0.57142857 -0.55714286 -0.54285714 -0.52857143 -0.51428571 -0.5 -0.48571429 -0.47142857 -0.45714286 -0.44285714 -0.42857143 -0.41428571 -0.4 -0.38571429 -0.37142857 -0.35714286 -0.34285714 -0.32857143 -0.31428571 -0.3 -0.28571429 -0.27142857 -0.25714286 -0.24285714 -0.22857143 -0.21428571 -0.2 -0.18571429 -0.17142857 -0.15714286 -0.14285714 -0.12857143 -0.11428571 -0.1 -0.08571429 -0.07142857 -0.05714286 -0.04285714 -0.02857143 -0.01428571 0 0 0 0 0 0
  line L41 (23.3434, 2.6406) -> (22.8484, 2.585)
  arc A85 (22.2971, 3.0149) -> (22.8484, 2.585) centre (22.7926, 3.0819) ccw
  arc A86 (22.2971, 3.0149) -> (22.1088, 4.1773) centre (0, 0) ccw
  arc A87 (22.4963, 4.7592) -> (22.1088, 4.1773) centre (22.6001, 4.2701) ccw
  line L42 (22.4963, 4.7592) -> (22.9835, 4.8627)
  spline S40 degree 5 poles (22.9835, 4.8627) (22.9936, 4.8648) (23.0137, 4.8693) (23.0435, 4.8768) (23.083, 4.8882) (23.1318, 4.9044) (23.1803, 4.9219) (23.2286, 4.9403) (23.2767, 4.9592) (23.3248, 4.9784) (23.3728, 4.998) (23.4206, 5.0179) (23.4683, 5.0385) (23.5158, 5.0597) (23.5632, 5.0815) (23.6103, 5.104) (23.6573, 5.127) (23.7041, 5.1504) (23.7508, 5.1743) (23.7974, 5.1984) (23.8439, 5.223) (23.8903, 5.2479) (23.9365, 5.2732) (23.9826, 5.299) (24.0286, 5.3251) (24.0744, 5.3517) (24.1201, 5.3786) (24.1657, 5.4058) (24.2111, 5.4334) (24.2565, 5.4613) (24.3017, 5.4896) (24.3468, 5.5181) (24.3918, 5.547) (24.4367, 5.5763) (24.4814, 5.6058) (24.526, 5.6357) (24.5705, 5.6658) (24.6149, 5.6963) (24.6592, 5.727) (24.7034, 5.7581) (24.7474, 5.7894) (24.7913, 5.8211) (24.8351, 5.853) (24.8788, 5.8852) (24.9224, 5.9177) (24.9659, 5.9504) (25.0092, 5.9834) (25.0524, 6.0167) (25.0955, 6.0503) (25.1385, 6.0841) (25.1814, 6.1182) (25.2242, 6.1525) (25.2668, 6.1871) (25.3094, 6.222) (25.3518, 6.2571) (25.3941, 6.2925) (25.4363, 6.3281) (25.4784, 6.3639) (25.5203, 6.4) (25.5622, 6.4364) (25.6039, 6.4729) (25.6455, 6.5098) (25.687, 6.5468) (25.7284, 6.5841) (25.7696, 6.6216) (25.8108, 6.6594) (25.8518, 6.6974) (25.8927, 6.7356) (25.9335, 6.774) (25.9742, 6.8127) (26.0147, 6.8516) (26.0471, 6.8829) (26.0713, 6.9064) (26.0874, 6.9222) (26.0955, 6.9301) knots 0 0 0 0 0 0 0.01428571 0.02857143 0.04285714 0.05714286 0.07142857 0.08571429 0.1 0.11428571 0.12857143 0.14285714 0.15714286 0.17142857 0.18571429 0.2 0.21428571 0.22857143 0.24285714 0.25714286 0.27142857 0.28571429 0.3 0.31428571 0.32857143 0.34285714 0.35714286 0.37142857 0.38571429 0.4 0.41428571 0.42857143 0.44285714 0.45714286 0.47142857 0.48571429 0.5 0.51428571 0.52857143 0.54285714 0.55714286 0.57142857 0.58571429 0.6 0.61428571 0.62857143 0.64285714 0.65714286 0.67142857 0.68571429 0.7 0.71428571 0.72857143 0.74285714 0.75714286 0.77142857 0.78571429 0.8 0.81428571 0.82857143 0.84285714 0.85714286 0.87142857 0.88571429 0.9 0.91428571 0.92857143 0.94285714 0.95714286 0.97142857 0.98571429 1 1 1 1 1 1
  arc A88 (26.0955, 6.9301) -> (25.6891, 8.311) centre (0, 0) ccw
  spline S41 degree 5 poles (25.6891, 8.311) (25.678, 8.3132) (25.6559, 8.3177) (25.6228, 8.3244) (25.5787, 8.3332) (25.5235, 8.3439) (25.4684, 8.3544) (25.4133, 8.3646) (25.3582, 8.3745) (25.3031, 8.3842) (25.2481, 8.3937) (25.1931, 8.4029) (25.1381, 8.4118) (25.0831, 8.4205) (25.0282, 8.4289) (24.9733, 8.437) (24.9185, 8.4449) (24.8637, 8.4525) (24.8089, 8.4599) (24.7541, 8.467) (24.6994, 8.4738) (24.6447, 8.4803) (24.5901, 8.4865) (24.5355, 8.4925) (24.4809, 8.4982) (24.4264, 8.5036) (24.372, 8.5088) (24.3176, 8.5136) (24.2632, 8.5182) (24.2089, 8.5225) (24.1546, 8.5265) (24.1004, 8.5302) (24.0462, 8.5336) (23.9921, 8.5367) (23.938, 8.5395) (23.884, 8.5419) (23.8301, 8.5441) (23.7762, 8.546) (23.7224, 8.5476) (23.6686, 8.5488) (23.615, 8.5497) (23.5613, 8.5503) (23.5078, 8.5506) (23.4543, 8.5505) (23.4009, 8.5501) (23.3476, 8.5493) (23.2944, 8.5482) (23.2412, 8.5468) (23.1882, 8.545) (23.1352, 8.5429) (23.0823, 8.5403) (23.0295, 8.5374) (22.9768, 8.5341) (22.9242, 8.5303) (22.8717, 8.5262) (22.8194, 8.5216) (22.7671, 8.5167) (22.7149, 8.5114) (22.6628, 8.5058) (22.6109, 8.4997) (22.5591, 8.493) (22.5075, 8.4857) (22.4561, 8.4778) (22.4049, 8.4692) (22.3538, 8.4601) (22.3029, 8.4505) (22.2521, 8.4406) (22.2014, 8.4304) (22.1509, 8.4198) (22.1006, 8.4082) (22.0508, 8.3954) (22.0115, 8.3836) (21.9823, 8.3737) (21.963, 8.3666) (21.9534, 8.363) knots -1 -1 -1 -1 -1 -1 -0.98571429 -0.97142857 -0.95714286 -0.94285714 -0.92857143 -0.91428571 -0.9 -0.88571429 -0.87142857 -0.85714286 -0.84285714 -0.82857143 -0.81428571 -0.8 -0.78571429 -0.77142857 -0.75714286 -0.74285714 -0.72857143 -0.71428571 -0.7 -0.68571429 -0.67142857 -0.65714286 -0.64285714 -0.62857143 -0.61428571 -0.6 -0.58571429 -0.57142857 -0.55714286 -0.54285714 -0.52857143 -0.51428571 -0.5 -0.48571429 -0.47142857 -0.45714286 -0.44285714 -0.42857143 -0.41428571 -0.4 -0.38571429 -0.37142857 -0.35714286 -0.34285714 -0.32857143 -0.31428571 -0.3 -0.28571429 -0.27142857 -0.25714286 -0.24285714 -0.22857143 -0.21428571 -0.2 -0.18571429 -0.17142857 -0.15714286 -0.14285714 -0.12857143 -0.11428571 -0.1 -0.08571429 -0.07142857 -0.05714286 -0.04285714 -0.02857143 -0.01428571 0 0 0 0 0 0
  line L43 (21.9534, 8.363) -> (21.4877, 8.186)
  arc A89 (20.8468, 8.4653) -> (21.4877, 8.186) centre (21.3101, 8.6534) ccw
  arc A90 (20.8468, 8.4653) -> (20.3754, 9.5443) centre (0, 0) ccw
  arc A91 (20.6059, 10.2043) -> (20.3754, 9.5443) centre (20.8282, 9.7564) ccw
  line L44 (20.6059, 10.2043) -> (21.0522, 10.4257)
  spline S42 degree 5 poles (21.0522, 10.4257) (21.0614, 10.4303) (21.0797, 10.4396) (21.1068, 10.4543) (21.1422, 10.4752) (21.1854, 10.503) (21.228, 10.532) (21.2702, 10.5619) (21.3121, 10.5921) (21.3539, 10.6227) (21.3955, 10.6535) (21.4369, 10.6848) (21.478, 10.7165) (21.5188, 10.7488) (21.5592, 10.7818) (21.5992, 10.8153) (21.639, 10.8492) (21.6785, 10.8836) (21.7179, 10.9183) (21.757, 10.9533) (21.7959, 10.9886) (21.8346, 11.0243) (21.8731, 11.0603) (21.9113, 11.0967) (21.9493, 11.1335) (21.9871, 11.1706) (22.0247, 11.208) (22.0621, 11.2457) (22.0993, 11.2838) (22.1362, 11.3221) (22.173, 11.3607) (22.2096, 11.3996) (22.246, 11.4388) (22.2822, 11.4782) (22.3182, 11.518) (22.354, 11.558) (22.3896, 11.5983) (22.425, 11.6388) (22.4602, 11.6796) (22.4953, 11.7207) (22.5301, 11.762) (22.5648, 11.8035) (22.5993, 11.8454) (22.6336, 11.8874) (22.6678, 11.9297) (22.7017, 11.9722) (22.7355, 12.015) (22.7691, 12.058) (22.8025, 12.1012) (22.8357, 12.1447) (22.8688, 12.1884) (22.9017, 12.2323) (22.9344, 12.2764) (22.9669, 12.3207) (22.9992, 12.3653) (23.0314, 12.41) (23.0634, 12.455) (23.0953, 12.5002) (23.1269, 12.5456) (23.1584, 12.5912) (23.1897, 12.637) (23.2209, 12.683) (23.2519, 12.7292) (23.2827, 12.7756) (23.3133, 12.8222) (23.3438, 12.869) (23.3741, 12.916) (23.4042, 12.9632) (23.4341, 13.0106) (23.4639, 13.0582) (23.4935, 13.1059) (23.5171, 13.1443) (23.5347, 13.1731) (23.5464, 13.1924) (23.5522, 13.202) knots 0 0 0 0 0 0 0.01428571 0.02857143 0.04285714 0.05714286 0.07142857 0.08571429 0.1 0.11428571 0.12857143 0.14285714 0.15714286 0.17142857 0.18571429 0.2 0.21428571 0.22857143 0.24285714 0.25714286 0.27142857 0.28571429 0.3 0.31428571 0.32857143 0.34285714 0.35714286 0.37142857 0.38571429 0.4 0.41428571 0.42857143 0.44285714 0.45714286 0.47142857 0.48571429 0.5 0.51428571 0.52857143 0.54285714 0.55714286 0.57142857 0.58571429 0.6 0.61428571 0.62857143 0.64285714 0.65714286 0.67142857 0.68571429 0.7 0.71428571 0.72857143 0.74285714 0.75714286 0.77142857 0.78571429 0.8 0.81428571 0.82857143 0.84285714 0.85714286 0.87142857 0.88571429 0.9 0.91428571 0.92857143 0.94285714 0.95714286 0.97142857 0.98571429 1 1 1 1 1 1
  arc A92 (23.5522, 13.202) -> (22.8151, 14.4385) centre (0, 0) ccw
  spline S43 degree 5 poles (22.8151, 14.4385) (22.8039, 14.4379) (22.7814, 14.4368) (22.7476, 14.435) (22.7027, 14.4326) (22.6466, 14.4292) (22.5906, 14.4256) (22.5347, 14.4218) (22.4788, 14.4178) (22.4231, 14.4135) (22.3674, 14.4089) (22.3119, 14.4042) (22.2564, 14.3991) (22.201, 14.3939) (22.1457, 14.3883) (22.0905, 14.3826) (22.0355, 14.3766) (21.9805, 14.3703) (21.9256, 14.3638) (21.8708, 14.357) (21.8161, 14.35) (21.7615, 14.3428) (21.707, 14.3352) (21.6527, 14.3274) (21.5984, 14.3194) (21.5443, 14.3111) (21.4902, 14.3025) (21.4363, 14.2937) (21.3825, 14.2846) (21.3288, 14.2752) (21.2753, 14.2656) (21.2218, 14.2557) (21.1685, 14.2455) (21.1153, 14.2351) (21.0623, 14.2243) (21.0094, 14.2133) (20.9566, 14.202) (20.9039, 14.1904) (20.8514, 14.1785) (20.799, 14.1664) (20.7468, 14.1539) (20.6947, 14.1412) (20.6428, 14.1281) (20.5911, 14.1147) (20.5394, 14.101) (20.488, 14.087) (20.4367, 14.0727) (20.3856, 14.0581) (20.3346, 14.0432) (20.2838, 14.028) (20.2332, 14.0124) (20.1828, 13.9964) (20.1326, 13.9801) (20.0826, 13.9633) (20.0328, 13.9463) (19.9832, 13.9288) (19.9338, 13.9111) (19.8846, 13.893) (19.8355, 13.8746) (19.7867, 13.8557) (19.7382, 13.8364) (19.6901, 13.8165) (19.6422, 13.7961) (19.5948, 13.775) (19.5476, 13.7535) (19.5007, 13.7315) (19.4539, 13.7093) (19.4073, 13.6868) (19.361, 13.6639) (19.3152, 13.6403) (19.2702, 13.6154) (19.235, 13.5942) (19.2092, 13.5774) (19.1923, 13.5657) (19.1839, 13.5598) knots -1 -1 -1 -1 -1 -1 -0.98571429 -0.97142857 -0.95714286 -0.94285714 -0.92857143 -0.91428571 -0.9 -0.88571429 -0.87142857 -0.85714286 -0.84285714 -0.82857143 -0.81428571 -0.8 -0.78571429 -0.77142857 -0.75714286 -0.74285714 -0.72857143 -0.71428571 -0.7 -0.68571429 -0.67142857 -0.65714286 -0.64285714 -0.62857143 -0.61428571 -0.6 -0.58571429 -0.57142857 -0.55714286 -0.54285714 -0.52857143 -0.51428571 -0.5 -0.48571429 -0.47142857 -0.45714286 -0.44285714 -0.42857143 -0.41428571 -0.4 -0.38571429 -0.37142857 -0.35714286 -0.34285714 -0.32857143 -0.31428571 -0.3 -0.28571429 -0.27142857 -0.25714286 -0.24285714 -0.22857143 -0.21428571 -0.2 -0.18571429 -0.17142857 -0.15714286 -0.14285714 -0.12857143 -0.11428571 -0.1 -0.08571429 -0.07142857 -0.05714286 -0.04285714 -0.02857143 -0.01428571 0 0 0 0 0 0
  line L45 (19.1839, 13.5598) -> (18.7769, 13.2726)
  arc A93 (18.0866, 13.3837) -> (18.7769, 13.2726) centre (18.4886, 13.6811) ccw
  arc A94 (18.0866, 13.3837) -> (17.3617, 14.3116) centre (0, 0) ccw
  arc A95 (17.4209, 15.0082) -> (17.3617, 14.3116) centre (17.7475, 14.6296) ccw
  line L46 (17.4209, 15.0082) -> (17.798, 15.3336)
  spline S44 degree 5 poles (17.798, 15.3336) (17.8058, 15.3403) (17.8212, 15.3539) (17.8438, 15.3749) (17.8729, 15.4039) (17.9079, 15.4416) (17.9419, 15.4803) (17.9753, 15.5197) (18.0084, 15.5595) (18.0413, 15.5994) (18.0739, 15.6397) (18.1062, 15.6802) (18.1382, 15.7212) (18.1696, 15.7627) (18.2005, 15.8046) (18.231, 15.847) (18.2611, 15.8898) (18.2908, 15.9329) (18.3203, 15.9763) (18.3495, 16.0199) (18.3784, 16.0638) (18.407, 16.108) (18.4353, 16.1525) (18.4633, 16.1972) (18.491, 16.2423) (18.5184, 16.2876) (18.5455, 16.3332) (18.5723, 16.3791) (18.5988, 16.4251) (18.6251, 16.4714) (18.6511, 16.518) (18.6769, 16.5647) (18.7024, 16.6117) (18.7276, 16.659) (18.7526, 16.7064) (18.7773, 16.7541) (18.8018, 16.8019) (18.826, 16.85) (18.85, 16.8983) (18.8737, 16.9468) (18.8972, 16.9955) (18.9205, 17.0444) (18.9435, 17.0934) (18.9663, 17.1427) (18.9888, 17.1921) (19.0111, 17.2418) (19.0332, 17.2916) (19.055, 17.3416) (19.0766, 17.3918) (19.098, 17.4421) (19.1192, 17.4927) (19.1401, 17.5434) (19.1608, 17.5942) (19.1813, 17.6453) (19.2016, 17.6965) (19.2216, 17.7478) (19.2414, 17.7994) (19.261, 17.8511) (19.2804, 17.9029) (19.2995, 17.9549) (19.3185, 18.0071) (19.3372, 18.0594) (19.3557, 18.1118) (19.374, 18.1644) (19.3921, 18.2172) (19.41, 18.2701) (19.4276, 18.3232) (19.4451, 18.3763) (19.4623, 18.4297) (19.4793, 18.4832) (19.4961, 18.5368) (19.5094, 18.5798) (19.5193, 18.6121) (19.5258, 18.6337) (19.5291, 18.6445) knots 0 0 0 0 0 0 0.01428571 0.02857143 0.04285714 0.05714286 0.07142857 0.08571429 0.1 0.11428571 0.12857143 0.14285714 0.15714286 0.17142857 0.18571429 0.2 0.21428571 0.22857143 0.24285714 0.25714286 0.27142857 0.28571429 0.3 0.31428571 0.32857143 0.34285714 0.35714286 0.37142857 0.38571429 0.4 0.41428571 0.42857143 0.44285714 0.45714286 0.47142857 0.48571429 0.5 0.51428571 0.52857143 0.54285714 0.55714286 0.57142857 0.58571429 0.6 0.61428571 0.62857143 0.64285714 0.65714286 0.67142857 0.68571429 0.7 0.71428571 0.72857143 0.74285714 0.75714286 0.77142857 0.78571429 0.8 0.81428571 0.82857143 0.84285714 0.85714286 0.87142857 0.88571429 0.9 0.91428571 0.92857143 0.94285714 0.95714286 0.97142857 0.98571429 1 1 1 1 1 1
  arc A96 (19.5291, 18.6445) -> (18.5077, 19.6588) centre (0, 0) ccw
  spline S45 degree 5 poles (18.5077, 19.6588) (18.4969, 19.6554) (18.4754, 19.6487) (18.4431, 19.6386) (18.4002, 19.6251) (18.3467, 19.6079) (18.2934, 19.5905) (18.2401, 19.5729) (18.1871, 19.5551) (18.1341, 19.537) (18.0814, 19.5188) (18.0287, 19.5004) (17.9763, 19.4817) (17.9239, 19.4628) (17.8717, 19.4437) (17.8197, 19.4244) (17.7679, 19.4049) (17.7162, 19.3852) (17.6646, 19.3652) (17.6132, 19.345) (17.562, 19.3246) (17.5109, 19.304) (17.46, 19.2832) (17.4093, 19.2621) (17.3588, 19.2408) (17.3084, 19.2193) (17.2582, 19.1976) (17.2082, 19.1756) (17.1583, 19.1534) (17.1086, 19.131) (17.0592, 19.1084) (17.0099, 19.0855) (16.9608, 19.0624) (16.9119, 19.039) (16.8631, 19.0154) (16.8146, 18.9916) (16.7663, 18.9675) (16.7182, 18.9432) (16.6703, 18.9186) (16.6226, 18.8938) (16.5751, 18.8688) (16.5278, 18.8435) (16.4808, 18.8179) (16.434, 18.7921) (16.3874, 18.766) (16.341, 18.7396) (16.2949, 18.713) (16.249, 18.6862) (16.2033, 18.659) (16.1579, 18.6316) (16.1128, 18.6039) (16.0679, 18.5759) (16.0234, 18.5476) (15.9791, 18.519) (15.9351, 18.4901) (15.8914, 18.4609) (15.848, 18.4314) (15.8048, 18.4016) (15.7619, 18.3716) (15.7193, 18.3412) (15.6771, 18.3104) (15.6354, 18.2792) (15.5942, 18.2475) (15.5534, 18.2153) (15.5131, 18.1827) (15.4731, 18.1498) (15.4334, 18.1166) (15.3938, 18.0832) (15.3547, 18.0495) (15.3162, 18.0152) (15.2788, 17.98) (15.25, 17.9507) (15.2292, 17.928) (15.2156, 17.9125) (15.209, 17.9046) knots -1 -1 -1 -1 -1 -1 -0.98571429 -0.97142857 -0.95714286 -0.94285714 -0.92857143 -0.91428571 -0.9 -0.88571429 -0.87142857 -0.85714286 -0.84285714 -0.82857143 -0.81428571 -0.8 -0.78571429 -0.77142857 -0.75714286 -0.74285714 -0.72857143 -0.71428571 -0.7 -0.68571429 -0.67142857 -0.65714286 -0.64285714 -0.62857143 -0.61428571 -0.6 -0.58571429 -0.57142857 -0.55714286 -0.54285714 -0.52857143 -0.51428571 -0.5 -0.48571429 -0.47142857 -0.45714286 -0.44285714 -0.42857143 -0.41428571 -0.4 -0.38571429 -0.37142857 -0.35714286 -0.34285714 -0.32857143 -0.31428571 -0.3 -0.28571429 -0.27142857 -0.25714286 -0.24285714 -0.22857143 -0.21428571 -0.2 -0.18571429 -0.17142857 -0.15714286 -0.14285714 -0.12857143 -0.11428571 -0.1 -0.08571429 -0.07142857 -0.05714286 -0.04285714 -0.02857143 -0.01428571 0 0 0 0 0 0
  line L47 (15.209, 17.9046) -> (14.8862, 17.5252)
  arc A97 (14.19, 17.4612) -> (14.8862, 17.5252) centre (14.5054, 17.8492) ccw
  arc A98 (14.19, 17.4612) -> (13.2571, 18.1796) centre (0, 0) ccw
  arc A99 (13.1412, 18.8691) -> (13.2571, 18.1796) centre (13.5517, 18.5836) ccw
  line L48 (13.1412, 18.8691) -> (13.4255, 19.2781)